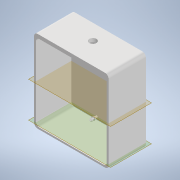
# Autodesk Inventor part: Part2
Saved by Autodesk Inventor 2022 (Build 260153000, 153)
## iProperties
Created: 2022-04-07
Part Number: Part2
Material: Generic
Document SubType Name: Modeling
Designer: Fred
Density: 1 g/cm^3
Appearance: Default
Author: Fred
Autodesk Inventor part; units mm, degrees
ref_plane "YZ Plane" through (0, 0, 0) normal (1, 0, 0) x (0, 1, 0)
ref_plane "XZ Plane" through (0, 0, 0) normal (0, 1, 0) x (-1, 0, 0)
ref_plane "XY Plane" through (0, 0, 0) normal (0, 0, 1) x (1, 0, 0)
sketch "Sketch1" plane through (0, 0, 0) normal (0, 0, 1) x (1, 0, 0)
  line L0 (0, 0) -> (66.04, 0)
  line L1 (66.04, 0) -> (66.04, 71.12)
  line L2 (66.04, 71.12) -> (0, 71.12)
  line L3 (0, 71.12) -> (0, 0)
  dimension "d0" = 71.12
  dimension "d1" = 66.04
  constraints: 8 end point, 2 parallel, 1 horizontal, 1 perpendicular
  measures "d0" distance of L0.end L1.end
  measures "d1" distance of L1.end L2.end
extrude "Extrusion1" add sketch "Sketch1" along normal blind 33.02
shell "Shell1" thickness 1.6 removed faces 1 at (44.0267, 23.7067, 33.02)
sketch "Sketch5" plane through (1.6, 69.52, 1.6) normal (0, 0, 1) x (1, 0, 0)
  circle A0 centre (22.53, -10.135) radius 1.1 projected
  circle A1 centre (22.53, -65.38) radius 1.25 projected
  circle A2 centre (40.31, -65.38) radius 1.25 projected
  point P0 (-1.6, -69.52)
  constraints: 3 coincident
ref_plane "Work Plane2" through (24.13, 4.14, 1.6) normal (0, -1, 0) x (1, 0, 0)
sketch "Sketch2" plane through (0, 71.12, 0) normal (0, 1, 0) x (1, 0, 0)
  line L0 (66.04, -33.02) -> (0, -33.02) projected
  line L1 (66.04, 0) -> (0, 0) projected
  point P0 (33.02, -13.97)
  point P1 (33.02, -13.97)
  point P2 (33.02, 0)
  dimension "d12" = 19.05
  constraints: 1 coincident, 1 midpoint, 1 vertical alignment
  measures "d12" distance from line of L0 point (33.02, -13.97)
hole "Hole1" at (33.02, 71.12, 13.97) direction (0, -1, 0) diameter 6.35 depth 1.6 tip angle 118
thicken "Thicken1" operation add thickness 1.6 both sides no extend neighbours yes toward (0, 1, 0) faces at (33.02, 71.12, 27.7283)
ref_plane "Work Plane1" through (1.6, 35.56, 1.6) normal (0, 1, 0) x (1, 0, 0)
sketch "Sketch3" plane through (1.6, 4.14, 1.6) normal (0, 1, 0) x (1, 0, 0)
  line L0 (0, 0) -> (62.84, 0) projected
  line L1 (64.44, 1.6) -> (-1.6, 1.6) projected
  line L2 (24.054, 0) -> (24.054, -3.048)
  line L3 (24.054, -3.048) -> (23.292, -3.048)
  line L4 (23.292, -3.048) -> (23.292, -4.972)
  line L5 (23.292, -4.972) -> (23.8508, -4.972)
  line L6 (23.8508, -4.972) -> (22.53, -6.8043)
  line L7 (22.53, -6.8043) -> (22.53, 0)
  line L8 (23.78, -4.775) -> (21.28, -4.775) projected
  line L9 (23.78, -4.775) -> (21.28, -4.775) projected
  line L10 (23.78, -4.775) -> (21.28, -4.775) projected
  line L11 (22.53, 0) -> (24.054, 0)
  point P0 (22.53, -4.775)
  dimension "d20" = 0.762
  dimension "d21" = 1.524
  dimension "d22" = 1.3208
  dimension "d30" = 3.048
  constraints: 14 end point, 3 perpendicular, 2 point on line, 1 collinear, 1 midpoint, 1 vertical alignment
  measures "d20" distance of L2.end L3.end
  measures "d21" distance between parallel lines of L7 L2
  measures "d22" distance from line of L7 L5.end
  measures "d30" distance between parallel lines of L0 L3
revolve "Revolution1" add sketch "Sketch3" angle 360 about axis through (24.13, 4.14, 8.4043) along (0, 0, -1)
fillet "Fillet1" radius 0.254 1 edges at (22.606, 4.14, 1.6)
sketch "Sketch4" plane through (1.6, 69.52, 4.648) normal (0, 0, 1) x (1, 0, 0)
  circle A0 centre (22.53, -65.38) radius 1.524 projected
  circle A1 centre (22.53, -65.38) radius 0.762 projected
  line L0 (20.4335, -65.0422) -> (24.6265, -65.0422)
  line L1 (24.6265, -65.0422) -> (24.6265, -65.7178)
  line L2 (24.6265, -65.7178) -> (20.4335, -65.7178)
  line L3 (20.4335, -65.7178) -> (20.4335, -65.0422)
  line L4 (20.4335, -65.0422) -> (24.6265, -65.7178) construction
  line L5 (24.6265, -65.0422) -> (20.4335, -65.7178) construction
  point P0 (-1.6, -69.52)
  constraints: 12 end point, 2 midpoint, 2 parallel, 1 horizontal, 1 perpendicular
extrude "Extrusion2" cut sketch "Sketch4" along normal blind 25.4 contours A0 L2 A1 L0 | A0 L0 L1 L2 | L0 A1 L2 A0 | A0 L2 L3 L0 | A1 L2 L0
pattern_sketch "Sketch Driven Pattern1" of "Revolution1", "Fillet1", "Extrusion2" from (24.13, 4.14, 1.6) copies at (41.91, 4.14, 1.6) at (24.13, 59.385, 1.6)
fillet "Fillet2" radius 3.175 8 edges at (0, 0, 16.51) (1.6, 1.6, 17.31) (1.6, 69.52, 17.31) (0, 72.72, 16.51) (66.04, 72.72, 16.51) (64.44, 69.52, 17.31) (66.04, 0, 16.51) (64.44, 1.6, 17.31)
sketch "Sketch6" plane through (3.175, 0, 0) normal (0, -1, 0) x (1, 0, 0)
  line L0 (26.884, 6.375) -> (25.884, 7.375) projected
  line L1 (32.684, 6.375) -> (26.884, 6.375) projected
  line L2 (33.684, 7.375) -> (32.684, 6.375) projected
  line L3 (33.684, 7.375) -> (33.684, 9.325) projected
  line L4 (25.884, 9.325) -> (33.684, 9.325) projected
  line L5 (25.884, 7.375) -> (25.884, 9.325) projected
  line L6 (25.2326, 9.9569) -> (34.6426, 9.9569)
  line L7 (34.6426, 9.9569) -> (34.6426, 5.4164)
  line L8 (34.6426, 5.4164) -> (25.2326, 5.4164)
  line L9 (25.2326, 5.4164) -> (25.2326, 9.9569)
  point P0 (-3.175, 0)
  constraints: 8 end point, 2 parallel, 1 horizontal, 1 perpendicular
extrude "Extrusion3" cut sketch "Sketch6" against normal blind 25.4 contours L0 L5 L4 L3 L2 L1 | L6 L7 L8 L9
chamfer "Chamfer1" distance 1.27 angle 45 1 edges at (33.1126, 0, 9.9569)
body "Solid1"
